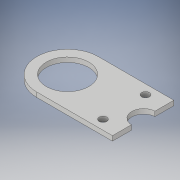
# Autodesk Inventor part: motor connector
Saved by Autodesk Inventor 2018 (Build 220112000, 112)
## iProperties
Created: 2019-01-23
Part Number: motor connector
Material: Generic
Document SubType Name: Modeling
Designer: s-2513225
Density: 1 g/cm^3
Appearance: Default
Author: s-2513225
Autodesk Inventor part; units mm, degrees
ref_plane "YZ Plane" through (0, 0, 0) normal (1, 0, 0) x (0, 1, 0)
ref_plane "XZ Plane" through (0, 0, 0) normal (0, 1, 0) x (-1, 0, 0)
ref_plane "XY Plane" through (0, 0, 0) normal (0, 0, 1) x (1, 0, 0)
sketch "Sketch1" plane through (0, 0, 0) normal (0, 1, 0) x (-1, 0, 0)
  circle A0 centre (0, 0) radius 14.2875
  arc A1 (0, -20.6375) -> (0, 20.6375) centre (0, 0) ccw
  line L0 (0, 20.6375) -> (-50.8, 20.6375)
  line L1 (0, -20.6375) -> (-50.8, -20.6375)
  line L2 (-50.8, -20.6375) -> (-50.8, -7.9375)
  line L3 (-50.8, 20.6375) -> (-50.8, 7.9375)
  arc A2 (-50.8, -7.9375) -> (-50.8, 7.9375) centre (-51.136, 0) ccw
  line L4 (-50.8, 14.2875) -> (-38.1, 14.2875) construction
  line L5 (-50.8, -14.2875) -> (-38.1, -14.2875) construction
  circle A3 centre (-38.1, -14.2875) radius 2.5797
  circle A4 centre (-38.1, 14.2875) radius 2.5797
  dimension "d0" = 28.575
  dimension "d1" = 6.35
  dimension "d2" = 50.8
  dimension "d3" = 50.8
  dimension "d4" = 12.7
  dimension "d5" = 12.7
  dimension "d6" = 12.7
  dimension "d7" = 5.1594
  dimension "d8" = 5.1594
  constraints: 12 end point, 5 centre point, 4 horizontal, 4 point on circle, 3 coincident, 2 midpoint, 2 tangent, 1 perpendicular, 1 vertical
  measures "d0" diameter of A0
  measures "d1" radial gap between concentric circles of A0 A1
  measures "d2" distance of L0.start L0.end
  measures "d3" distance of L1.start L1.end
  measures "d4" distance of L1.end L2.end
  measures "d5" distance of L0.end L3.end
  measures "d6" distance of L4.start L4.end
  measures "d7" diameter of A3
  measures "d8" diameter of A4
extrude "Extrusion1" add sketch "Sketch1" along normal blind 3.175
body "Solid1"
